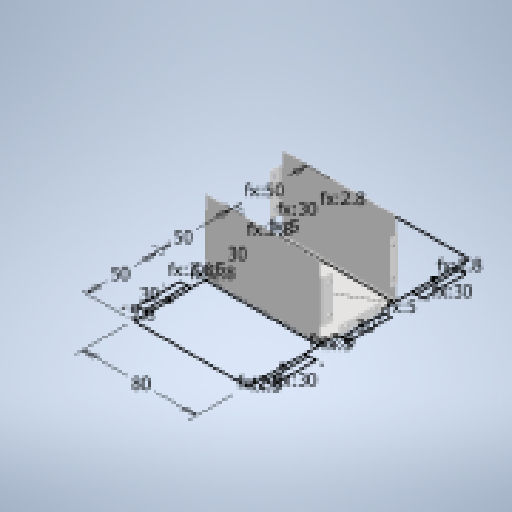
# Autodesk Inventor part: Bottom
Saved by Autodesk Inventor 2024 (Build 280153000, 153)
## iProperties
Created: 2025-10-28
Part Number: Bottom
Material: 일반
Document SubType Name: Sheet Metal
Designer: alexi
Density: 1 g/cm^3
Sheet Metal Rule: 기본값_mm
Appearance: 기본값
Author: alexi
Autodesk Inventor part; units mm, degrees
ref_plane "YZ Plane" through (0, 0, 0) normal (1, 0, 0) x (0, 1, 0)
ref_plane "XZ Plane" through (0, 0, 0) normal (0, 1, 0) x (-1, 0, 0)
ref_plane "XY Plane" through (0, 0, 0) normal (0, 0, 1) x (1, 0, 0)
sketch "스케치1" plane through (0, 0, 0) normal (0, 1, 0) x (-1, 0, 0)
  line L0 (40, -25) -> (-40, -25)
  line L1 (-40, -25) -> (-40, 25)
  line L2 (-40, 25) -> (40, 25)
  line L3 (40, 25) -> (40, -25)
  line L4 (40, -25) -> (-40, -25)
  line L5 (-40, -25) -> (-40, -27.8)
  line L6 (-40, -27.8) -> (40, -27.8)
  line L7 (40, -27.8) -> (40, -25)
  line L8 (40, 25) -> (-40, 25)
  line L9 (-40, 25) -> (-40, 27.8)
  line L10 (-40, 27.8) -> (40, 27.8)
  line L11 (40, 27.8) -> (40, 25)
  line L12 (40, 27.8) -> (-40, 27.8)
  line L13 (-40, 27.8) -> (-40, 77.8)
  line L14 (-40, 77.8) -> (40, 77.8)
  line L15 (40, 77.8) -> (40, 27.8)
  line L16 (40, -27.8) -> (-40, -27.8)
  line L17 (-40, -27.8) -> (-40, -77.8)
  line L18 (-40, -77.8) -> (40, -77.8)
  line L19 (40, -77.8) -> (40, -27.8)
  line L20 (40, 25) -> (-40, -25) construction
  line L21 (40, -25) -> (-40, 25) construction
  line L22 (40, 26.4) -> (-40, 26.4) construction
  line L23 (40, -26.4) -> (-40, -26.4) construction
  line L24 (40, -15) -> (42.8, -15)
  line L25 (42.8, -15) -> (42.8, 15)
  line L26 (42.8, 15) -> (40, 15)
  line L27 (40, 15) -> (40, -15)
  line L28 (-40, -15) -> (-42.8, -15)
  line L29 (-42.8, -15) -> (-42.8, 15)
  line L30 (-42.8, 15) -> (-40, 15)
  line L31 (-40, 15) -> (-40, -15)
  line L32 (42.8, -15) -> (47.8, -15)
  line L33 (47.8, -15) -> (47.8, 15)
  line L34 (47.8, 15) -> (42.8, 15)
  line L35 (42.8, 15) -> (42.8, -15)
  line L36 (-42.8, -15) -> (-47.8, -15)
  line L37 (-47.8, -15) -> (-47.8, 15)
  line L38 (-47.8, 15) -> (-42.8, 15)
  line L39 (-42.8, 15) -> (-42.8, -15)
  line L40 (40, -67.8) -> (42.8, -67.8)
  line L41 (42.8, -67.8) -> (42.8, -37.8)
  line L42 (42.8, -37.8) -> (40, -37.8)
  line L43 (40, -37.8) -> (40, -67.8)
  line L44 (-40, -67.8) -> (-42.8, -67.8)
  line L45 (-42.8, -67.8) -> (-42.8, -37.8)
  line L46 (-42.8, -37.8) -> (-40, -37.8)
  line L47 (-40, -37.8) -> (-40, -67.8)
  line L48 (40, 37.8) -> (42.8, 37.8)
  line L49 (42.8, 37.8) -> (42.8, 67.8)
  line L50 (42.8, 67.8) -> (40, 67.8)
  line L51 (40, 67.8) -> (40, 37.8)
  line L52 (42.8, 37.8) -> (47.8, 37.8)
  line L53 (47.8, 37.8) -> (47.8, 67.8)
  line L54 (47.8, 67.8) -> (42.8, 67.8)
  line L55 (42.8, 67.8) -> (42.8, 37.8)
  line L56 (-42.8, -67.8) -> (-47.8, -67.8)
  line L57 (-47.8, -67.8) -> (-47.8, -37.8)
  line L58 (-47.8, -37.8) -> (-42.8, -37.8)
  line L59 (-42.8, -37.8) -> (-42.8, -67.8)
  line L60 (42.8, -67.8) -> (47.8, -67.8)
  line L61 (47.8, -67.8) -> (47.8, -37.8)
  line L62 (47.8, -37.8) -> (42.8, -37.8)
  line L63 (42.8, -37.8) -> (42.8, -67.8)
  line L64 (-40, 37.8) -> (-42.8, 37.8)
  line L65 (-42.8, 37.8) -> (-42.8, 67.8)
  line L66 (-42.8, 67.8) -> (-40, 67.8)
  line L67 (-40, 67.8) -> (-40, 37.8)
  line L68 (-42.8, 37.8) -> (-47.8, 37.8)
  line L69 (-47.8, 37.8) -> (-47.8, 67.8)
  line L70 (-47.8, 67.8) -> (-42.8, 67.8)
  line L71 (-42.8, 67.8) -> (-42.8, 37.8)
  point P0 (0, 0)
  point P1 (0, 0)
  point P2 (40, 0)
  point P3 (-40, 0)
  point P4 (-40, 15)
  point P5 (40, 15)
  point P6 (40, -52.8)
  point P7 (-40, -52.8)
  point P8 (40, 52.8)
  point P9 (-40, 52.8)
  point P10 (-40, -37.8)
  point P11 (-40, 67.8)
  point P12 (40, 67.8)
  dimension "d0" = 50
  dimension "d1" = 80
  dimension "d2" = 2.8
  dimension "d3" = 2.8
  dimension "d4" = 50
  dimension "d5" = 50
  dimension "d19" = 30
  dimension "d20" = 30
  dimension "d21" = 2.8
  dimension "d22" = 2.8
  dimension "d23" = 5
  dimension "d24" = 5
  dimension "d37" = 2.8
  dimension "d38" = 2.8
  dimension "d40" = 2.8
  dimension "d41" = 5
  dimension "d43" = 5
  dimension "d44" = 5
  dimension "d45" = 2.8
  dimension "d46" = 5
  dimension "d47" = 30
  dimension "d48" = 30
  dimension "d49" = 30
  dimension "d50" = 30
  constraints: 144 end point, 34 parallel, 18 midpoint, 17 horizontal, 17 perpendicular, 10 point on line, 1 coincident
  measures "d0" distance of L2.end L0.start
  measures "d1" distance of L13.end L14.end
  measures "d2" distance of L10.end L2.end
  measures "d3" distance of L6.end L0.start
  measures "d4" distance of L14.end L10.end
  measures "d5" distance of L18.end L6.end
  measures "d19" distance of L24.end L25.end
  measures "d20" distance of L28.end L29.end
  measures "d21" distance of L25.end L26.end
  measures "d22" distance of L29.end L30.end
  measures "d23" distance of L25.end L33.end
  measures "d24" distance of L29.end L37.end
  measures "d37" distance of L40.start L40.end
  measures "d38" distance of L44.start L44.end
  measures "d40" distance of L49.end L50.end
  measures "d41" distance of L49.end L53.end
  measures "d43" distance of L41.end L61.end
  measures "d44" distance of L45.end L57.end
  measures "d45" distance of L65.end L66.end
  measures "d46" distance of L69.end L65.end
  measures "d47" distance of L52.end L53.end
  measures "d48" distance of L68.end L69.end
  measures "d49" distance of L60.end L61.end
  measures "d50" distance of L56.end L57.end
extrude "판1" add sketch "스케치1" against normal blind 0.5
fold "접기11" angle 90 bend radius 1.5 thickness 0.5 k factor 0.44 line from (42.8, 0, 37.8) to (42.8, 0, 67.8) line at bend end moving side (1, 0, 0) folds toward (0, 1, 0)
fold "접기12" angle 90 bend radius 1.5 thickness 0.5 k factor 0.44 line from (-42.8, 0, 37.8) to (-42.8, 0, 67.8) line at bend end moving side (-1, 0, 0) folds toward (0, 1, 0)
fold "접기13" angle 90 bend radius 1.5 thickness 0.5 k factor 0.44 line from (42.8, 0, -15) to (42.8, 0, 15) line at bend end moving side (1, 0, 0) folds toward (0, 1, 0)
fold "접기14" angle 90 bend radius 1.5 thickness 0.5 k factor 0.44 line from (-42.8, 0, -15) to (-42.8, 0, 15) line at bend end moving side (-1, 0, 0) folds toward (0, 1, 0)
fold "접기15" angle 90 bend radius 1.5 thickness 0.5 k factor 0.44 line from (42.8, 0, -37.8) to (42.8, 0, -67.8) line at bend end moving side (1, 0, 0) folds toward (0, 1, 0)
fold "접기16" angle 90 bend radius 1.5 thickness 0.5 k factor 0.44 line from (-42.8, 0, -67.8) to (-42.8, 0, -37.8) line at bend end moving side (-1, 0, 0) folds toward (0, 1, 0)
fold "접기17" angle 90 bend radius 1.5 thickness 0.5 k factor 0.44 line from (40, 0, 27.8) to (-40, 0, 27.8) line at bend end moving side (0, 0, 1) folds toward (0, 1, 0)
fold "접기18" angle 90 bend radius 1.5 thickness 0.5 k factor 0.44 line from (40, 0, -27.8) to (-40, 0, -27.8) line at bend end moving side (0, 0, -1) folds toward (0, 1, 0)
sketch "스케치3" plane through (-42.0982, 11.5, -20.0982) normal (-1, 0, 0) x (0, 0, 1)
  line L0 (45.1965, 0) -> (45.1965, 30) projected
  line L1 (40.1965, 30) -> (45.1965, 30) projected
  line L2 (40.1965, 0) -> (40.1965, 30) projected
  line L3 (45.1965, 0) -> (40.1965, 0) projected
  line L4 (-5, 30) -> (-5, 0) projected
  line L5 (0, 0) -> (-5, 0) projected
  line L6 (0, 30) -> (0, 0) projected
  line L7 (-5, 30) -> (0, 30) projected
  line L8 (5.0982, -10) -> (35.0982, -10) projected
  line L9 (35.0982, -5) -> (35.0982, -10) projected
  line L10 (5.0982, -5) -> (35.0982, -5) projected
  line L11 (5.0982, -10) -> (5.0982, -5) projected
  line L12 (-2.5, 30) -> (-2.5, 0) construction
  line L13 (42.6965, 30) -> (42.6965, 0) construction
  line L14 (5.0982, -7.5) -> (35.0982, -7.5) construction
  point P0 (20.0982, -11.5)
  point P1 (-2.5, 5)
  point P2 (-2.5, 25)
  point P3 (10.0982, -7.5)
  point P4 (30.0982, -7.5)
  point P5 (42.6965, 5)
  point P6 (42.6965, 25)
  dimension "d135" = 5
  dimension "d136" = 5
  dimension "d137" = 5
  dimension "d138" = 5
  dimension "d139" = 5
  dimension "d140" = 5
  constraints: 6 end point, 6 midpoint, 6 point on line
  measures "d135" distance from line of L5 point (-2.5, 5)
  measures "d136" distance from line of L7 point (-2.5, 25)
  measures "d137" distance from line of L11 point (10.098, -7.5)
  measures "d138" distance from line of L9 point (30.098, -7.5)
  measures "d139" distance from line of L3 point (42.696, 5)
  measures "d140" distance from line of L1 point (42.696, 25)
hole "구멍1" at (-42.0982, 16.5, -22.5982) at (-42.0982, 4, -10) at (-42.0982, 4, 10) at (-42.0982, 16.5, 22.5982) at (-42.0982, 36.5, 22.5982) at (-42.0982, 36.5, -22.5982) direction (1, 0, 0) diameter 2.459 depth 0.5 tip angle 118 thread size "M3x0.5" class "6H" standard "ANSI Metric M Profile"
sketch "스케치4" plane through (42.0982, 11.5, 20.0982) normal (1, 0, 0) x (0, 0, -1)
  line L0 (-5, 30) -> (-5, 0) projected
  line L1 (0, 0) -> (-5, 0) projected
  line L2 (0, 30) -> (0, 0) projected
  line L3 (-5, 30) -> (0, 30) projected
  line L4 (5.0982, -10) -> (35.0982, -10) projected
  line L5 (35.0982, -5) -> (35.0982, -10) projected
  line L6 (5.0982, -5) -> (35.0982, -5) projected
  line L7 (5.0982, -10) -> (5.0982, -5) projected
  line L8 (45.1965, 0) -> (45.1965, 30) projected
  line L9 (40.1965, 30) -> (45.1965, 30) projected
  line L10 (40.1965, 0) -> (40.1965, 30) projected
  line L11 (45.1965, 0) -> (40.1965, 0) projected
  line L12 (-2.5, 30) -> (-2.5, 0) construction
  line L13 (5.0982, -10) -> (5.0982, -5) projected
  line L14 (5.0982, -7.5) -> (35.0982, -7.5) construction
  line L15 (42.6965, 0) -> (42.6965, 30) construction
  point P0 (20.0982, -11.5)
  point P1 (-2.5, 25)
  point P2 (-2.5, 5)
  point P3 (10.0982, -7.5)
  point P4 (30.0982, -7.5)
  point P5 (42.6965, 25)
  point P6 (42.6965, 5)
  dimension "d148" = 5
  dimension "d149" = 5
  dimension "d150" = 5
  dimension "d151" = 5
  dimension "d152" = 5
  dimension "d153" = 5
  constraints: 6 end point, 6 midpoint, 6 point on line
  measures "d148" distance from line of point (-2.5, 25) L3
  measures "d149" distance from line of L1 point (-2.5, 5)
  measures "d150" distance from line of L7 point (10.098, -7.5)
  measures "d151" distance from line of L5 point (30.098, -7.5)
  measures "d152" distance from line of L11 point (42.696, 5)
  measures "d153" distance from line of L9 point (42.696, 25)
hole "구멍2" at (42.0982, 36.5, 22.5982) at (42.0982, 16.5, 22.5982) at (42.0982, 4, 10) at (42.0982, 4, -10) at (42.0982, 16.5, -22.5982) at (42.0982, 36.5, -22.5982) direction (-1, 0, 0) diameter 2.459 depth 0.5 tip angle 118 thread size "M3x0.5" class "6H" standard "ANSI Metric M Profile"
equation "\"d2\" = d40"
equation "\"d3\" = d40"
equation "\"d5\" = d4"
equation "\"d21\" = d40"
equation "\"d22\" = d40"
equation "\"d23\" = d41"
equation "\"d24\" = d41"
equation "\"d37\" = d40"
equation "\"d38\" = d40"
equation "\"d43\" = d41"
equation "\"d44\" = d41"
equation "\"d45\" = d40"
equation "\"d46\" = d41"
equation "\"d48\" = d47"
equation "\"d49\" = d47"
equation "\"d50\" = d47"
equation "\"d87\" = BendReliefWidth"
equation "\"d88\" = BendReliefDepth"
equation "\"d89\" = MinimumRemnant"
equation "\"d90\" = TransitionRadius"
equation "\"d93\" = BendReliefWidth"
equation "\"d94\" = BendReliefDepth"
equation "\"d95\" = MinimumRemnant"
equation "\"d96\" = TransitionRadius"
equation "\"d99\" = BendReliefWidth"
equation "\"d100\" = BendReliefDepth"
equation "\"d101\" = MinimumRemnant"
equation "\"d102\" = TransitionRadius"
equation "\"d105\" = BendReliefWidth"
equation "\"d106\" = BendReliefDepth"
equation "\"d107\" = MinimumRemnant"
equation "\"d108\" = TransitionRadius"
equation "\"d111\" = BendReliefWidth"
equation "\"d112\" = BendReliefDepth"
equation "\"d113\" = MinimumRemnant"
equation "\"d114\" = TransitionRadius"
equation "\"d117\" = BendReliefWidth"
equation "\"d118\" = BendReliefDepth"
equation "\"d119\" = MinimumRemnant"
equation "\"d120\" = TransitionRadius"
equation "\"d123\" = BendReliefWidth"
equation "\"d124\" = BendReliefDepth"
equation "\"d125\" = MinimumRemnant"
equation "\"d126\" = TransitionRadius"
equation "\"d129\" = BendReliefWidth"
equation "\"d130\" = BendReliefDepth"
equation "\"d131\" = MinimumRemnant"
equation "\"d132\" = TransitionRadius"
equation "\"TransitionRadius\" = BendRadius"
equation "\"BendReliefWidth\" = 0.5"
equation "\"BendReliefDepth\" = 0.25"
equation "\"MinimumRemnant\" = 1"
equation "\"BendRadius\" = 0.5"
